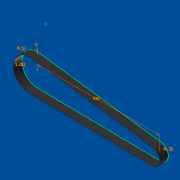
# Autodesk Inventor part: Szij
Saved by Autodesk Inventor 2015 SP1 (Build 190203100, 203)
## iProperties
Created: 2014-10-26
Part Number: Szij
Material: Generic
Document SubType Name: Modeling
Designer: laca
Density: 1 g/cm^3
Appearance: Default
Mass: 46.9557 g
Surface Area: 762.78 cm^2
Volume: 46.9557 cm^3
Author: laca
Autodesk Inventor part; units mm, degrees
ref_plane "YZ Plane" through (0, 0, 0) normal (1, 0, 0) x (0, 1, 0)
ref_plane "XZ Plane" through (0, 0, 0) normal (0, 1, 0) x (-1, 0, 0)
ref_plane "XY Plane" through (0, 0, 0) normal (0, 0, 1) x (1, 0, 0)
sketch "Sketch1" plane through (0, 0, 0) normal (0, 0, 1) x (1, 0, 0)
  arc A0 (-22.5975, -105.4525) -> (-31.0052, -218.9372) centre (-30.2027, -161.9428) ccw
  arc A1 (419.3749, -225.2787) -> (423.8, -165.5499) centre (419.7973, -195.2817) ccw
  line L0 (-22.5975, -105.4525) -> (423.8, -165.5499)
  line L1 (-31.0052, -218.9372) -> (419.3749, -225.2787)
  arc A2 (-22.4265, -104.1818) -> (-31.0232, -220.2191) centre (-30.2027, -161.9428) ccw
  line L2 (-22.4265, -104.1818) -> (423.9711, -164.2793)
  arc A3 (419.3569, -226.5607) -> (423.9711, -164.2793) centre (419.7973, -195.2817) ccw
  line L3 (419.3569, -226.5607) -> (-31.0232, -220.2191)
  arc A4 (-27.7033, -103.7144) -> (-32.7021, -103.7144) centre (-30.2027, -103.6607) ccw
  point P0 (0, 0)
  dimension "d1" = 57
  dimension "d2" = 30
  dimension "d3" = 450
  dimension "d4" = 1.2821
  dimension "d7" = 5
  constraints: 13 point on circle, 8 end point, 5 centre point, 4 tangent, 3 other
  measures "d1" radius of A0
  measures "d2" radius of A1
  measures "d3" horizontal distance of A1.centre A0.centre
  measures "d4" radial gap between concentric circles of A2 A0
  measures "d7" diameter of A4
extrude "Extrusion1" add sketch "Sketch1" along normal blind 31 contours L2 A3 L3 A2
sketch "Sketch2" plane through (0, 0, 0) normal (0, 0, -1) x (-1, 0, 0)
  point P0 (0, 0)
extrude "Extrusion3" [suppressed]
equation "\"d1\" = 0.5 * NagyKerekAtmero"
equation "\"d2\" = 0.5 * KisKerekAtmero"
equation "\"d5\" = SzíjSzélességA"
equation "\"NagyKerekAtmero\" = 114"
equation "\"KisKerekAtmero\" = 60"
equation "\"SzíjSzélességA\" = 31"
body "Solid1"
